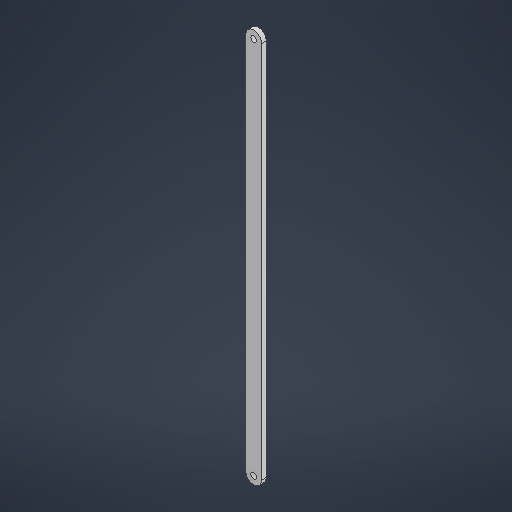
# Autodesk Inventor part: RedKangoroo_003_bar3ipt
Saved by Autodesk Inventor 2026.3 (Build 303398000, 398)
## iProperties
Created: 2026-05-22
Part Number: RedKangoroo_003_bar3ipt
Material: Generic
Document SubType Name: Modeling
Designer: ADMIN
Density: 1 g/cm^3
Appearance: Default
Author: ADMIN
Autodesk Inventor part; units mm, degrees
ref_plane "YZ Plane" through (0, 0, 0) normal (1, 0, 0) x (0, 1, 0)
ref_plane "XZ Plane" through (0, 0, 0) normal (0, 1, 0) x (-1, 0, 0)
ref_plane "XY Plane" through (0, 0, 0) normal (0, 0, 1) x (1, 0, 0)
sketch "Sketch1" plane through (0, 0, 0) normal (0, 0, 1) x (1, 0, 0)
  line L0 (0, 0) -> (0, 240.36) construction
  line L1 (0, 0) -> (240.36, 0) construction
  circle A0 centre (0, 0) radius 1.75
  circle A1 centre (0, 240.36) radius 1.75
  line L2 (0, 240.36) -> (0, 0) construction
  line L3 (-5, 240.36) -> (-5, 0)
  line L4 (5, 0) -> (5, 240.36)
  arc A2 (5, 240.36) -> (-5, 240.36) centre (0, 240.36) ccw
  arc A3 (-5, 0) -> (5, 0) centre (0, 0) ccw
  point P0 (0, 120.18)
  point P1 (0, 120.18)
  dimension "d0" = 240.36
  dimension "d1" = 90
  dimension "d3" = 3.5
  dimension "d4" = 3.5
  dimension "d7" = 10
  constraints: 14 end point, 4 centre point, 4 point on circle, 4 tangent, 2 coincident, 2 midpoint, 2 perpendicular, 1 horizontal, 1 parallel, 1 vertical
  measures "d0" distance of L0.start L0.end
  measures "d1" angle of L1 L0
  measures "d3" diameter of A0
  measures "d4" diameter of A1
  measures "d7" diameter of A3
extrude "Extrusion2" add sketch "Sketch1" along normal blind 3
body "Solid2"
